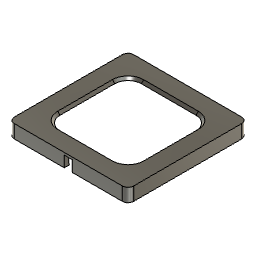
key frame (Autodesk Fusion 360 design; units mm, degrees)
Autodesk Fusion 360 part; units mm, degrees
sketch "Sketch1" plane through (0, 0, 0) normal (0, 0, 1) x (1, 0, 0)
  line L0 (0.2, 0) -> (16.4, 0)
  line L1 (16.6, 0.2) -> (16.6, 16.4)
  line L2 (16.4, 16.6) -> (0.2, 16.6)
  line L3 (0, 16.4) -> (0, 0.2)
  arc A0 (0.2, 16.6) -> (0, 16.4) centre (0.2, 16.4) ccw
  arc A1 (16.6, 16.4) -> (16.4, 16.6) centre (16.4, 16.4) ccw
  arc A2 (16.4, 0) -> (16.6, 0.2) centre (16.4, 0.2) ccw
  arc A3 (0, 0.2) -> (0.2, 0) centre (0.2, 0.2) ccw
  line L4 (16.4, 17.25) -> (0.2, 17.25)
  arc A4 (0.2, 17.25) -> (-0.65, 16.4) centre (0.2, 16.4) ccw
  line L5 (-0.65, 16.4) -> (-0.65, 0.2)
  arc A5 (-0.65, 0.2) -> (0.2, -0.65) centre (0.2, 0.2) ccw
  line L6 (0.2, -0.65) -> (16.4, -0.65)
  arc A6 (16.4, -0.65) -> (17.25, 0.2) centre (16.4, 0.2) ccw
  line L7 (17.25, 0.2) -> (17.25, 16.4)
  arc A7 (17.25, 16.4) -> (16.4, 17.25) centre (16.4, 16.4) ccw
  line L8 (14.4, 14.4) -> (2.2, 14.4)
  line L9 (2.2, 14.4) -> (2.2, 2.2)
  line L10 (2.2, 2.2) -> (14.4, 2.2)
  line L11 (14.4, 2.2) -> (14.4, 14.4)
  line L12 (0.2, -5) -> (16.4, -5)
  arc A8 (16.4, -5) -> (21.6, 0.2) centre (16.4, 0.2) ccw
  line L13 (21.6, 0.2) -> (21.6, 16.4)
  arc A9 (21.6, 16.4) -> (16.4, 21.6) centre (16.4, 16.4) ccw
  line L14 (16.4, 21.6) -> (0.2, 21.6)
  arc A10 (0.2, 21.6) -> (-5, 16.4) centre (0.2, 16.4) ccw
  line L15 (-5, 16.4) -> (-5, 0.2)
  arc A11 (-5, 0.2) -> (0.2, -5) centre (0.2, 0.2) ccw
  point P0 (16.6, 0)
  point P1 (0, 16.6)
  dimension "d1" = 16.6
  dimension "d2" = 16.6
  dimension "d3" = 0.2
  dimension "d4" = 0.65
  dimension "d5" = -2.2
  dimension "d15" = 5
  constraint horizontal L0
  constraint vertical L1
  constraint horizontal L2
  constraint vertical L3
  constraint coincident P1 L2
  constraint coincident P1 L3
  constraint tangent L2 A0
  constraint tangent L3 A0
  constraint tangent L1 A1
  constraint tangent L2 A1
  constraint equal A0 A1
  constraint coincident P0 L0
  constraint coincident P0 L1
  constraint tangent L0 A2
  constraint tangent L1 A2
  constraint equal A0 A2
  constraint coincident origin L0
  constraint coincident origin L3
  constraint tangent L0 A3
  constraint tangent L3 A3
  constraint equal A0 A3
  measures "d1" distance of origin P0
  measures "d2" distance of origin P1
  measures "d3" radius of A0
extrude "Extrude1" add sketch "Sketch1" along normal blind 0.35 contours L0 L1 L2 L3 A0 A1 A2 A3 | L4 A4 L5 A5 L6 A6 L7 A7
extrude "Extrude2" add sketch "Sketch1" against normal blind 1.35 contours L4 A4 L5 A5 L6 A6 L7 A7
fillet "Fillet1" radius 2 4 edges at (2.2, 14.4, 0.175) (14.4, 14.4, 0.175) (14.4, 2.2, 0.175) (2.2, 2.2, 0.175)
chamfer "Chamfer1" distance 0.35 angle 45 8 edges at (8.3, 14.4, 0.35) (13.8142, 13.8142, 0.35) (14.4, 8.3, 0.35) (13.8142, 2.7858, 0.35) (8.3, 2.2, 0.35) (2.7858, 2.7858, 0.35) (2.2, 8.3, 0.35) (2.7858, 13.8142, 0.35)
extrude "Extrude3" add 1 faces at (17.0333, 5.6, -1.35) along direction (0, 0, -1) blind 0.3 draft 30
extrude "Extrude4" cut sketch "Sketch1" against normal blind 6 contours L12 A8 L13 A9 L14 A10 L15 A11
chamfer "Chamfer2" distance 0.1 angle 45 8 edges at (8.3, 16.4268, -1.65) (0.1811, 16.4189, -1.65) (0.1732, 8.3, -1.65) (0.1811, 0.1811, -1.65) (8.3, 0.1732, -1.65) (16.4189, 0.1811, -1.65) (16.4268, 8.3, -1.65) (16.4189, 16.4189, -1.65)
sketch "Sketch2" plane through (0, 0, -1.65) normal (0, 0, -1) x (1, 0, 0)
  line L0 (17.25, -16.4) -> (17.25, -0.2)
  arc A0 (17.25, -0.2) -> (16.4, 0.65) centre (16.4, -0.2) ccw
  line L1 (16.4, 0.65) -> (0.2, 0.65)
  arc A1 (0.2, 0.65) -> (-0.65, -0.2) centre (0.2, -0.2) ccw
  line L2 (-0.65, -0.2) -> (-0.65, -16.4)
  arc A2 (-0.65, -16.4) -> (0.2, -17.25) centre (0.2, -16.4) ccw
  line L3 (0.2, -17.25) -> (16.4, -17.25)
  arc A3 (16.4, -17.25) -> (17.25, -16.4) centre (16.4, -16.4) ccw
  line L4 (16.4, -16.5268) -> (0.2, -16.5268)
  arc A4 (0.0732, -16.4) -> (0.2, -16.5268) centre (0.2, -16.4) ccw
  line L5 (0.0732, -16.4) -> (0.0732, -0.2)
  arc A5 (0.2, -0.0732) -> (0.0732, -0.2) centre (0.2, -0.2) ccw
  line L6 (0.2, -0.0732) -> (16.4, -0.0732)
  arc A6 (16.5268, -0.2) -> (16.4, -0.0732) centre (16.4, -0.2) ccw
  line L7 (16.5268, -0.2) -> (16.5268, -16.4)
  arc A7 (16.4, -16.5268) -> (16.5268, -16.4) centre (16.4, -16.4) ccw
  line L8 (8.3, 0.65) -> (8.3, -17.25) construction
  line L9 (7.7, -17.25) -> (7.7, 0.65)
  line L10 (8.9, -17.25) -> (8.9, 0.65)
  line L11 (8.3, -8.3) -> (0.2, 0.65)
  line L12 (8.3, -8.3) -> (-0.65, -0.2)
  line L13 (8.3, -8.3) -> (-0.65, -16.4)
  line L14 (8.3, -8.3) -> (0.2, -17.25)
  line L15 (8.3, -8.3) -> (16.4, -17.25)
  line L16 (8.3, -8.3) -> (17.25, -16.4)
  line L17 (8.3, -8.3) -> (17.25, -0.2)
  line L18 (8.3, -8.3) -> (16.4, 0.65)
  point P0 (0.5, -16.2)
  point P1 (0.5, -0.5)
  point P2 (16.2, -0.5)
  point P3 (16.2, -16.2)
  dimension "d19" = 0.6
  dimension "d23" = 360
  constraint midpoint L1 L8.start
  constraint midpoint L3 L8.end
  constraint coincident L3 L9.start
  constraint coincident L1 L9.end
  constraint perpendicular L1 L9
  constraint symmetric L8 L9.start L10.start
  constraint symmetric L8 L9.end L10.end
  constraint midpoint L8 L11.start
  constraint coincident L1.end A1.start
  constraint coincident A1.end L2.start
  measures "d19" distance of L8 L9
extrude "Extrude5" cut sketch "Sketch2" against normal up to surface (1.65 mm away) contours L3 L4 L9 L10 | L1 L6 L9 L10 | L4 L9 L10 L14 L15 | L6 L9 L10 L11 L18
equation "d1 = d2"
